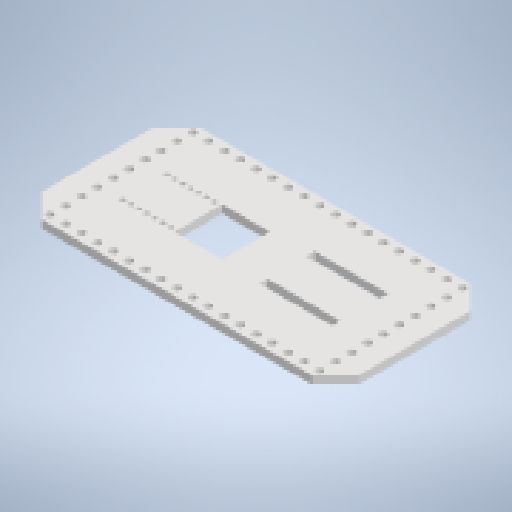
# Autodesk Inventor part: Chasis1
Saved by Autodesk Inventor 2024 (Build 280153000, 153)
## iProperties
Created: 2024-03-25
Part Number: Chasis1
Material: Generic
Document SubType Name: Modeling
Designer: JDAM
Density: 1 g/cm^3
Appearance: Default
Author: JDAM
Autodesk Inventor part; units mm, degrees
ref_plane "YZ Plane" through (0, 0, 0) normal (1, 0, 0) x (0, 1, 0)
ref_plane "XZ Plane" through (0, 0, 0) normal (0, 1, 0) x (-1, 0, 0)
ref_plane "XY Plane" through (0, 0, 0) normal (0, 0, 1) x (1, 0, 0)
sketch "Sketch1" plane through (0, 0, 0) normal (0, 1, 0) x (-1, 0, 0)
  line L0 (-100, 50) -> (100, 50)
  line L1 (100, 50) -> (100, -50)
  line L2 (100, -50) -> (-100, -50)
  line L3 (-100, -50) -> (-100, 50)
  line L4 (-100, 50) -> (100, -50) construction
  line L5 (100, 50) -> (-100, -50) construction
  point P0 (0, 0)
  dimension "d0" = 200
  dimension "d1" = 100
  constraints: 12 end point, 2 midpoint, 2 parallel, 1 horizontal, 1 perpendicular
  measures "d0" distance of L1.end L2.end
  measures "d1" distance of L0.end L1.end
extrude "Extrusion1" add sketch "Sketch1" along normal blind 5
chamfer "Chamfer1" distance 15 angle 45 4 edges at (100, 2.5, -50) (100, 2.5, 50) (-100, 2.5, 50) (-100, 2.5, -50)
sketch "Sketch2" plane through (0, 5, 0) normal (0, 1, 0) x (1, 0, 0)
  line L0 (-85, -50) -> (85, -50) projected
  line L1 (85, 50) -> (85, -50)
  line L2 (85, 0) -> (0, 0)
  line L3 (85, 50) -> (-85, 50) projected
  line L4 (85, 0) -> (75, 0)
  line L5 (75, 0) -> (75, 50)
  line L6 (85, -50) -> (85, -45)
  line L7 (85, -45) -> (87.1749, -45)
  dimension "d7" = 10
  dimension "d15" = 5
  constraints: 12 end point, 3 point on line, 2 horizontal, 1 midpoint, 1 perpendicular, 1 vertical
  measures "d7" distance of L2.start L4.end
  measures "d15" distance of L0.end L6.end
hole "Hole2" at (85, 5, 45) direction (0, -1, 0) diameter 4.6 depth 12
pattern_linear "Rectangular Pattern1" count 10 spacing 10 along (0, 0, -1) of "Hole2"
mirror "Mirror1" about plane through (0, 0, 0) normal (1, 0, 0) of "Hole2", "Rectangular Pattern1"
sketch "Sketch4" plane through (0, 5, 0) normal (0, 1, 0) x (1, 0, 0)
  line L0 (-80.0603, -82.0418) -> (-80.0603, 17.9582)
  line L1 (90.6107, -82.0418) -> (90.6107, 17.9582)
  line L2 (-0.0013, -0.0056) -> (-0.0013, -50.0056)
  line L3 (83.0525, -0.0056) -> (83.0525, -82.0364)
  line L4 (83.0525, -0.0056) -> (-0.0013, -0.0056)
  line L5 (41.5256, -0.0056) -> (41.5256, -11.4056)
  line L6 (41.5256, -0.0056) -> (41.5256, 12.9944)
  line L7 (41.5256, 12.9944) -> (64.5256, 12.9944)
  line L8 (64.5256, 12.9944) -> (64.5256, -11.4056)
  line L9 (64.5256, -11.4056) -> (41.5256, -11.4056)
  line L10 (41.5256, -11.4056) -> (18.5256, -11.4056)
  line L11 (18.5256, -11.4056) -> (18.5256, 12.9944)
  line L12 (18.5256, 12.9944) -> (41.5256, 12.9944)
  line L13 (41.5256, 12.9944) -> (41.5256, 18.4944)
  line L14 (41.5256, 18.4944) -> (64.5256, 18.4944)
  line L15 (64.5256, 18.4944) -> (64.5256, 12.9944)
  line L16 (41.5256, 18.4944) -> (18.5256, 18.4944)
  line L17 (18.5256, 12.9944) -> (18.5256, 18.4944)
  line L18 (41.5256, -11.4056) -> (41.5256, -16.5056)
  line L19 (41.5256, -16.5056) -> (64.5256, -16.5056)
  line L20 (64.5256, -16.5056) -> (64.5256, -11.4056)
  line L21 (41.5256, -16.5056) -> (18.5256, -16.5056)
  line L22 (18.5256, -16.5056) -> (18.5256, -11.4056)
  point P0 (0, 0)
  dimension "d31" = 100
  dimension "d32" = 50
  dimension "d35" = 23
  dimension "d36" = 23
  dimension "d37" = 5.5
  dimension "d38" = 23
  dimension "d39" = 23
  dimension "d40" = 5.1
  dimension "d41" = 23
  dimension "d42" = 23
  dimension "d56" = 35
  constraints: 46 end point, 7 perpendicular, 6 vertical, 4 point on line, 2 horizontal, 1 collinear, 1 midpoint, 1 parallel
  measures "d31" distance of L0.start L0.end
  measures "d32" distance of L2.start L2.end
  measures "d35" distance of L6.end L7.end
  measures "d36" distance of L5.end L10.end
  measures "d37" distance of L6.end L13.end
  measures "d38" distance of L13.end L14.end
  measures "d39" distance of L13.end L16.end
  measures "d40" distance of L5.end L18.end
  measures "d41" distance of L18.end L19.end
  measures "d42" distance of L18.end L21.end
  measures "d56" distance of L21.end L16.end
extrude "Extrusion3" cut sketch "Sketch4" against normal blind 10 contours L7 L13 L14 L15 | L20 L19 L18 L9 | L18 L21 L22 L10 | L12 L17 L16 L13
sketch "Sketch6" plane through (0, 0, 0) normal (0, -1, 0) x (1, 0, 0)
  line L0 (100, 35) -> (100, -35) projected
  line L1 (100, 0) -> (-99.9985, 0)
  line L2 (0, 0) -> (-99.9985, 0)
  line L3 (-49.9993, 0) -> (-49.9993, 50)
  line L4 (-85, 50) -> (85, 50) projected
  line L5 (-49.9993, 0) -> (-49.9993, -50.9458)
  circle A0 centre (-50.1056, -13.7921) radius 1.5
  dimension "d70" = 3
  constraints: 8 end point, 2 midpoint, 2 point on line, 1 centre point, 1 collinear, 1 horizontal, 1 perpendicular
  measures "d70" diameter of A0
hole "Hole3" at (-50.1056, 0, -13.7921) direction (0, 1, 0) diameter 3 depth 12.7625
pattern_linear "Rectangular Pattern2" count 3 spacing 5 along (1, 0, 0) count 3 spacing 10 along (-1, 0, 0) of "Hole3"
mirror "Mirror2" about plane through (0, 0, 0) normal (0, 0, 1) of "Hole3", "Rectangular Pattern2"
sketch "Sketch7" plane through (0, 5, 0) normal (0, 1, 0) x (1, 0, 0)
  circle A0 centre (-85, -45) radius 2.3 projected
  line L0 (-85, -45) -> (-75, -45)
  circle A1 centre (-75, -45) radius 2.3
  point P0 (0, 0)
  dimension "d84" = 10
  dimension "d85" = 4.6
  constraints: 2 end point, 1 centre point, 1 coincident, 1 horizontal
  measures "d84" distance of L0.start L0.end
  measures "d85" diameter of A1
hole "Hole4" at (-75, 5, 45) direction (0, -1, 0) diameter 4.6 depth 7
pattern_linear "Rectangular Pattern3" count 16 spacing 10 along (1, 0, 0) of "Hole4"
mirror "Mirror3" about plane through (0, 0, 0) normal (0, 0, 1) of "Hole4", "Rectangular Pattern3"
sketch "Sketch8" plane through (0, 5, 0) normal (0, 1, 0) x (1, 0, 0)
  line L0 (-6.2494, -15) -> (-36.2494, -15)
  line L1 (-36.2494, -15) -> (-36.2494, 15)
  line L2 (-36.2494, 15) -> (-6.2494, 15)
  line L3 (-6.2494, 15) -> (-6.2494, -15)
  line L4 (-6.2494, -15) -> (-36.2494, 15) construction
  line L5 (-36.2494, -15) -> (-6.2494, 15) construction
  point P0 (0, 0)
  point P1 (-21.2494, 0)
  dimension "d96" = 30
  dimension "d97" = 30
  constraints: 12 end point, 2 midpoint, 2 parallel, 1 horizontal, 1 perpendicular
  measures "d96" distance of L1.end L2.end
  measures "d97" distance of L0.end L1.end
extrude "Extrusion5" cut sketch "Sketch8" against normal blind 10
body "Solid1"
